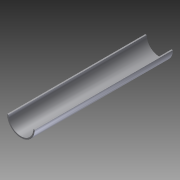
# Autodesk Inventor part: target
Saved by Autodesk Inventor 2012 (Build 160160000, 160)
## iProperties
Created: 2012-06-22
Part Number: target
Material: Default
Document SubType Name: Modeling
Designer: wberry
Density: 1 g/cm^3
Author: wberry
Autodesk Inventor part; units mm, degrees
ref_plane "YZ Plane" through (0, 0, 0) normal (1, 0, 0) x (0, 1, 0)
ref_plane "XZ Plane" through (0, 0, 0) normal (0, 1, 0) x (-1, 0, 0)
ref_plane "XY Plane" through (0, 0, 0) normal (0, 0, 1) x (1, 0, 0)
sketch "Sketch1" plane through (0, 0, 0) normal (0, 0, 1) x (1, 0, 0)
  circle A0 centre (0, 0) radius 50
  circle A1 centre (0, 0) radius 45
  line L0 (-50, 0) -> (-45, 0)
  line L1 (45, 0) -> (50, 0)
  dimension "d0" = 100
  dimension "d1" = 90
  constraints: 4 end point, 4 point on circle, 3 coincident, 2 centre point, 1 collinear, 1 horizontal
  measures "d0" diameter of A0
  measures "d1" diameter of A1
extrude "Extrusion1" add sketch "Sketch1" along normal blind 500 contours A0 L0 A1 L1 picked at (0, -46.5023)
body "Solid1"
